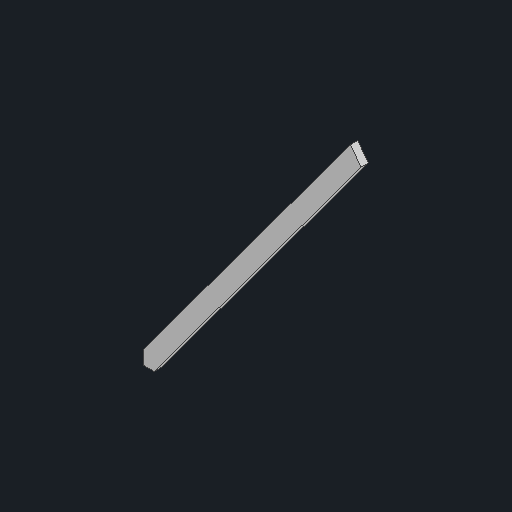
# Autodesk Inventor part: 74+
Saved by Autodesk Inventor 2026 (Build 300175000, 175)
## iProperties
Created: 2025-09-04
Part Number: 74+
Material: Generic
Document SubType Name: Modeling
Designer: trott
Density: 1 g/cm^3
Appearance: Default
Author: trott
Autodesk Inventor part; units mm, degrees
ref_plane "YZ Plane" through (0, 0, 0) normal (1, 0, 0) x (0, 1, 0)
ref_plane "XZ Plane" through (0, 0, 0) normal (0, 1, 0) x (-1, 0, 0)
ref_plane "XY Plane" through (0, 0, 0) normal (0, 0, 1) x (1, 0, 0)
sketch "Sketch1" plane through (0, 0, 0) normal (0, 0, 1) x (1, 0, 0)
  line L0 (-571.5, -1549.4) -> (571.5, -1549.4)
  line L1 (571.5, -1549.4) -> (571.5, 1549.4)
  line L2 (571.5, 1549.4) -> (-571.5, 1549.4)
  line L3 (-571.5, 1549.4) -> (-571.5, -1549.4)
  line L4 (-571.5, -1549.4) -> (571.5, 1549.4) construction
  line L5 (571.5, -1549.4) -> (-571.5, 1549.4) construction
  line L6 (-571.5, 0) -> (571.5, 0)
  line L7 (571.5, 0) -> (-571.5, -1549.4)
  line L8 (-535.73, -1575.7877) -> (-607.27, -1523.0123)
  line L9 (607.27, -26.3877) -> (535.73, 26.3877)
  line L10 (535.73, 26.3877) -> (-607.27, -1523.0123)
  line L11 (-535.73, -1575.7877) -> (607.27, -26.3877)
  line L12 (535.73, 26.3877) -> (571.5, 74.8759)
  line L13 (-571.5, 1549.4) -> (571.5, -1549.4) construction
  line L14 (571.5, 0) -> (-571.5, 1549.4)
  line L15 (-535.73, 1575.7877) -> (-607.27, 1523.0123)
  line L16 (607.27, 26.3877) -> (535.73, -26.3877)
  line L17 (535.73, -26.3877) -> (-607.27, 1523.0123)
  line L18 (-535.73, 1575.7877) -> (607.27, 26.3877)
  line L19 (535.73, -26.3877) -> (571.5, -74.8759)
  point P0 (0, 0)
  point P1 (571.5, 74.8759)
  point P2 (-516.2637, 1549.4)
  point P3 (-571.5, 1474.5241)
  point P4 (571.5, -74.8759)
  point P5 (571.5, -74.8759)
  point P6 (516.2637, 0)
  point P7 (-571.5, -1474.5241)
  point P8 (-516.2637, -1549.4)
  dimension "d0" = 1143
  dimension "d1" = 3098.8
  dimension "d3" = 88.9
  dimension "d4" = 88.9
  constraints: 40 end point, 6 midpoint, 5 symmetric about line, 3 perpendicular, 3 point on line, 2 parallel, 1 horizontal
  measures "d0" distance of L2.end L1.end
  measures "d1" distance of L0.end L1.end
  measures "d3" distance of L8.start L8.end
  measures "d4" distance of L9.start L9.end
extrude "Extrusion1" add sketch "Sketch1" along normal blind 38.1 contours L7 L19 L11 L0 | L3 L10 L17 L19 L7
body "Solid1"
